Autodesk Fusion 360 part; units mm, degrees
(part 2 of 13)
  line L913 (104.217, -70.819) -> (104.221, -70.8155)
  line L914 (88.0199, -70.6373) -> (87.9134, -70.4952)
  line L915 (87.7957, -72.4288) -> (87.4385, -72.4288)
  line L916 (87.2885, -70.2788) -> (87.3086, -70.2038)
  line L917 (108.814, -71.9394) -> (108.833, -71.9473)
  line L918 (104.14, -72.3538) -> (104.085, -72.4087)
  line L919 (87.5885, -72.1288) -> (87.7639, -72.1288)
  line L920 (88.0792, -71.7621) -> (88.1457, -71.4077)
  line L921 (104.296, -70.7954) -> (104.439, -70.7954)
  line L922 (104.01, -70.7954) -> (104.085, -70.8155)
  line L923 (104.286, -70.7957) -> (104.291, -70.7967)
  line L924 (104.085, -72.4087) -> (104.01, -72.4288)
  line L925 (104.514, -71.0753) -> (104.439, -71.0954)
  line L926 (87.5885, -70.4288) -> (87.5885, -72.1288)
  line L927 (88.1457, -71.1498) -> (88.0792, -70.7954)
  line L928 (104.221, -70.8155) -> (104.254, -70.8067)
  line L929 (87.3086, -72.3538) -> (87.2885, -72.2788)
  line L930 (104.257, -71.1512) -> (104.214, -71.2087)
  line L931 (104.214, -71.2087) -> (104.16, -71.3536)
  line L932 (87.4385, -72.4288) -> (87.3635, -72.4087)
  line L933 (104.139, -70.8696) -> (104.212, -70.8206)
  line L934 (108.805, -71.9407) -> (108.814, -71.9394)
  line L935 (87.3086, -70.2038) -> (87.3635, -70.1489)
  line L936 (108.886, -71.9683) -> (108.899, -71.9851)
  line L937 (108.899, -71.9851) -> (108.916, -71.9983)
  line L938 (108.987, -72.0935) -> (108.994, -72.1103)
  line L939 (87.4385, -70.1288) -> (87.7957, -70.1288)
  line L940 (88.2808, -72.0632) -> (88.2728, -72.083)
  line L941 (88.1457, -71.4077) -> (88.1457, -71.1498)
  line L942 (104.439, -71.0954) -> (104.341, -71.0954)
  line L943 (88.0199, -71.9202) -> (88.0792, -71.7621)
  line L944 (87.8566, -72.4158) -> (87.8258, -72.4207)
  line L945 (87.7957, -70.1288) -> (87.8258, -70.1368)
  line L946 (103.371, -70.8155) -> (103.426, -70.8704)
  line L947 (102.792, -72.4087) -> (102.789, -72.4052)
  line L948 (103.371, -72.4087) -> (103.296, -72.4288)
  line L949 (108.814, -72.4277) -> (108.805, -72.4264)
  line L950 (108.73, -71.956) -> (108.737, -71.9503)
  line L951 (108.877, -71.9649) -> (108.886, -71.9683)
  line L952 (108.758, -71.9473) -> (108.778, -71.9394)
  line L953 (108.778, -71.9394) -> (108.787, -71.9407)
  line L954 (109.008, -72.2213) -> (109.005, -72.2424)
  line L955 (108.604, -72.2735) -> (108.598, -72.2567)
  line L956 (108.721, -71.9584) -> (108.73, -71.956)
  line L957 (108.598, -72.1103) -> (108.604, -72.0935)
  line L958 (102.611, -72.2737) -> (102.59, -72.25)
  line L959 (108.871, -71.9584) -> (108.877, -71.9649)
  line L960 (108.787, -72.4264) -> (108.778, -72.4277)
  line L961 (108.787, -71.9407) -> (108.796, -71.9383)
  line L962 (108.604, -72.0935) -> (108.676, -71.9983)
  line L963 (108.586, -72.1246) -> (108.598, -72.1103)
  line L964 (109.005, -72.2424) -> (108.994, -72.2567)
  line L965 (108.862, -72.411) -> (108.855, -72.4167)
  line L966 (109.016, -72.2015) -> (109.008, -72.2213)
  line L967 (103.426, -70.8704) -> (103.446, -70.9454)
  line L968 (108.692, -72.382) -> (108.676, -72.3688)
  line L969 (108.586, -72.2424) -> (108.583, -72.2213)
  line L970 (108.833, -72.4197) -> (108.814, -72.4277)
  line L971 (108.862, -71.956) -> (108.871, -71.9584)
  line L972 (108.583, -72.2213) -> (108.575, -72.2015)
  line L973 (108.758, -72.4197) -> (108.737, -72.4167)
  line L974 (108.598, -72.2567) -> (108.586, -72.2424)
  line L975 (108.737, -71.9503) -> (108.758, -71.9473)
  line L976 (109.005, -72.1246) -> (109.008, -72.1458)
  line L977 (108.916, -71.9983) -> (108.987, -72.0935)
  line L978 (108.855, -72.4167) -> (108.833, -72.4197)
  line L979 (108.796, -72.4288) -> (108.787, -72.4264)
  line L980 (108.778, -72.4277) -> (108.758, -72.4197)
  line L981 (109.013, -72.1835) -> (109.016, -72.2015)
  line L982 (108.994, -72.2567) -> (108.987, -72.2735)
  line L983 (108.871, -72.4087) -> (108.862, -72.411)
  line L984 (108.721, -72.4087) -> (108.714, -72.4022)
  line L985 (108.706, -72.3988) -> (108.692, -72.382)
  line L986 (108.676, -71.9983) -> (108.692, -71.9851)
  line L987 (108.575, -72.1656) -> (108.583, -72.1458)
  line L988 (108.796, -71.9383) -> (108.805, -71.9407)
  line L989 (108.994, -72.1103) -> (109.005, -72.1246)
  line L990 (108.877, -72.4022) -> (108.871, -72.4087)
  line L991 (108.676, -72.3688) -> (108.604, -72.2735)
  line L992 (108.583, -72.1458) -> (108.586, -72.1246)
  line L993 (108.805, -72.4264) -> (108.796, -72.4288)
  line L994 (109.016, -72.1656) -> (109.013, -72.1835)
  line L995 (108.916, -72.3688) -> (108.899, -72.382)
  line L996 (108.855, -71.9503) -> (108.862, -71.956)
  line L997 (108.692, -71.9851) -> (108.706, -71.9683)
  line L998 (109.008, -72.1458) -> (109.016, -72.1656)
  line L999 (108.833, -71.9473) -> (108.855, -71.9503)
  line L1000 (108.706, -71.9683) -> (108.714, -71.9649)
  line L1001 (108.886, -72.3988) -> (108.877, -72.4022)
  line L1002 (108.714, -71.9649) -> (108.721, -71.9584)
  line L1003 (108.899, -72.382) -> (108.886, -72.3988)
  line L1004 (108.987, -72.2735) -> (108.916, -72.3688)
  line L1005 (108.575, -72.2015) -> (108.578, -72.1835)
  line L1006 (108.578, -72.1835) -> (108.575, -72.1656)
  line L1007 (108.73, -72.411) -> (108.721, -72.4087)
  line L1008 (108.737, -72.4167) -> (108.73, -72.411)
  line L1009 (108.714, -72.4022) -> (108.706, -72.3988)
  line L1010 (133.278, -90.9545) -> (133.338, -90.8098)
  line L1011 (135.594, -81.6495) -> (135.593, -81.6559)
  line L1012 (134.438, -90.9545) -> (134.458, -91.1098)
  line L1013 (133.963, -83.4223) -> (133.964, -83.425)
  line L1014 (133.606, -83.3536) -> (133.61, -83.3452)
  line L1015 (133.631, -83.2877) -> (133.638, -83.2823)
  line L1016 (135.348, -72.6427) -> (135.292, -72.6351)
  line L1017 (135.596, -81.647) -> (135.594, -81.6495)
  line L1018 (135.562, -81.7087) -> (133.908, -83.3628)
  line L1019 (133.61, -83.3452) -> (133.609, -83.3362)
  line L1020 (133.946, -83.4014) -> (133.96, -83.4192)
  line L1021 (133.858, -91.7098) -> (133.703, -91.6894)
  line L1022 (134.158, -91.6294) -> (134.013, -91.6894)
  line L1023 (134.892, -71.4334) -> (135.012, -71.3164)
  line L1024 (133.558, -91.6294) -> (133.434, -91.5341)
  line L1025 (133.908, -83.3628) -> (133.946, -83.4014)
  line L1026 (106.922, -87.5998) -> (106.862, -87.4551)
  line L1027 (133.278, -91.2651) -> (133.258, -91.1098)
  line L1028 (133.338, -91.4098) -> (133.278, -91.2651)
  line L1029 (135.598, -72.6444) -> (135.598, -81.6204)
  line L1030 (133.619, -83.4136) -> (133.614, -83.4064)
  line L1031 (133.733, -83.5416) -> (133.643, -83.4512)
  line L1032 (133.643, -83.4512) -> (133.621, -83.4224)
  line L1033 (134.013, -91.6894) -> (133.858, -91.7098)
  line L1034 (108.022, -87.1445) -> (108.042, -87.2998)
  line L1035 (106.862, -87.4551) -> (106.842, -87.2998)
  line L1036 (135.577, -81.6817) -> (135.562, -81.7087)
  line L1037 (134.378, -91.4098) -> (134.282, -91.5341)
  line L1038 (133.434, -91.5341) -> (133.338, -91.4098)
  line L1039 (133.338, -90.8098) -> (133.434, -90.6855)
  line L1040 (107.142, -87.8194) -> (107.018, -87.7241)
  line L1041 (135.154, -71.2288) -> (135.312, -71.1749)
  line L1042 (133.643, -83.2744) -> (135.348, -81.5686)
  line L1043 (134.438, -91.2651) -> (134.378, -91.4098)
  line L1044 (133.258, -91.1098) -> (133.278, -90.9545)
  line L1045 (133.96, -83.4192) -> (133.963, -83.4223)
  line L1046 (135.624, -72.6421) -> (135.598, -72.6444)
  line L1047 (133.622, -83.3127) -> (133.631, -83.2877)
  line L1048 (133.983, -90.5263) -> (134.013, -90.5302)
  line L1049 (135.783, -72.5904) -> (135.624, -72.6421)
  line L1050 (133.612, -83.3797) -> (133.606, -83.3536)
  line L1051 (134.378, -90.8098) -> (134.438, -90.9545)
  line L1052 (133.434, -90.6855) -> (133.558, -90.5902)
  line L1053 (133.609, -83.3362) -> (133.622, -83.3127)
  line L1054 (133.638, -83.2823) -> (133.643, -83.2744)
  line L1055 (133.558, -90.5902) -> (133.703, -90.5302)
  line L1056 (134.282, -91.5341) -> (134.158, -91.6294)
  line L1057 (135.292, -72.6351) -> (135.135, -72.5768)
  line L1058 (108.022, -87.4551) -> (107.962, -87.5998)
  line L1059 (107.742, -87.8194) -> (107.597, -87.8794)
  line L1060 (133.703, -91.6894) -> (133.558, -91.6294)
  line L1061 (133.964, -83.425) -> (133.968, -83.4302)
  line L1062 (133.614, -83.4064) -> (133.612, -83.3797)
  line L1063 (135.348, -81.5686) -> (135.348, -72.6427)
  line L1064 (108.042, -87.2998) -> (108.022, -87.4551)
  line L1065 (107.442, -87.8998) -> (107.287, -87.8794)
  line L1066 (135.312, -71.1749) -> (135.479, -71.1574)
  line L1067 (133.733, -90.5263) -> (133.733, -83.5416)
  line L1068 (133.621, -83.4224) -> (133.619, -83.4136)
  line L1069 (135.012, -71.3164) -> (135.154, -71.2288)
  line L1070 (134.74, -72.0633) -> (134.724, -71.8969)
  line L1071 (136.048, -72.3895) -> (135.927, -72.5048)
  line L1072 (136.2, -72.0939) -> (136.141, -72.2502)
  line L1073 (133.703, -90.5302) -> (133.733, -90.5263)
  line L1074 (107.866, -87.7241) -> (107.742, -87.8194)
  line L1075 (134.995, -72.4853) -> (134.879, -72.365)
  line L1076 (106.842, -87.2998) -> (106.862, -87.1445)
  line L1077 (128.608, -80.6108) -> (128.615, -80.6409)
  line L1078 (120.961, -72.2502) -> (120.869, -72.3895)
  line L1079 (107.597, -86.7202) -> (107.742, -86.7802)
  line L1080 (111.956, -87.6733) -> (111.831, -87.7686)
  line L1081 (120.764, -71.3229) -> (120.882, -71.4415)
  line L1082 (112.131, -87.249) -> (112.111, -87.4043)
  line L1083 (111.231, -86.7294) -> (111.376, -86.6694)
  line L1084 (107.018, -86.8755) -> (107.142, -86.7802)
  line L1085 (111.956, -86.8247) -> (112.051, -86.949)
  line L1086 (112.051, -87.549) -> (111.956, -87.6733)
  line L1087 (107.597, -87.8794) -> (107.442, -87.8998)
  line L1088 (106.862, -87.1445) -> (106.922, -86.9998)
  line L1089 (110.931, -87.249) -> (110.952, -87.0937)
  line L1090 (107.287, -87.8794) -> (107.142, -87.8194)
  line L1091 (106.922, -86.9998) -> (107.018, -86.8755)
  line L1092 (111.531, -87.849) -> (111.376, -87.8286)
  line L1093 (120.623, -71.2333) -> (120.764, -71.3229)
  line L1094 (111.107, -87.6733) -> (111.012, -87.549)
  line L1095 (112.111, -87.4043) -> (112.051, -87.549)
  line L1096 (107.962, -86.9998) -> (108.022, -87.1445)
  line L1097 (107.287, -86.7202) -> (107.442, -86.6998)
  line L1098 (112.111, -87.0937) -> (112.131, -87.249)
  line L1099 (107.742, -86.7802) -> (107.866, -86.8755)
  line L1100 (107.018, -87.7241) -> (106.922, -87.5998)
  line L1101 (135.135, -72.5768) -> (134.995, -72.4853)
  line L1102 (111.831, -87.7686) -> (111.687, -87.8286)
  line L1103 (120.466, -71.1772) -> (120.623, -71.2333)
  line L1104 (111.687, -87.8286) -> (111.531, -87.849)
  line L1105 (135.479, -71.1574) -> (135.645, -71.1772)
  line L1106 (107.866, -86.8755) -> (107.962, -86.9998)
  line L1107 (128.605, -80.6056) -> (128.608, -80.6108)
  line L1108 (128.615, -80.6409) -> (128.624, -80.6704)
  line L1109 (111.012, -86.949) -> (111.107, -86.8247)
  line L1110 (128.624, -86.7664) -> (128.621, -86.7846)
  line L1111 (128.621, -86.7846) -> (128.621, -86.7895)
  line L1112 (134.724, -71.8969) -> (134.744, -71.731)
  line L1113 (107.962, -87.5998) -> (107.866, -87.7241)
  line L1114 (111.376, -87.8286) -> (111.231, -87.7686)
  line L1115 (110.952, -87.0937) -> (111.012, -86.949)
  line L1116 (128.415, -87.0369) -> (128.447, -87.1)
  line L1117 (134.744, -71.731) -> (134.802, -71.5739)
  line L1118 (111.107, -86.8247) -> (111.231, -86.7294)
  line L1119 (111.831, -86.7294) -> (111.956, -86.8247)
  line L1120 (134.879, -72.365) -> (134.793, -72.222)
  line L1121 (112.051, -86.949) -> (112.111, -87.0937)
  line L1122 (107.142, -86.7802) -> (107.287, -86.7202)
  line L1123 (111.376, -86.6694) -> (111.531, -86.649)
  line L1124 (107.442, -86.6998) -> (107.597, -86.7202)
  line L1125 (128.447, -87.1) -> (128.467, -87.2236)
  line L1126 (128.621, -86.7895) -> (128.62, -86.7928)
  line L1127 (110.952, -87.4043) -> (110.931, -87.249)
  line L1128 (111.531, -86.649) -> (111.687, -86.6694)
  line L1129 (111.687, -86.6694) -> (111.831, -86.7294)
  line L1130 (128.467, -87.2236) -> (128.447, -87.3472)
  line L1131 (134.793, -72.222) -> (134.74, -72.0633)
  line L1132 (134.802, -71.5739) -> (134.892, -71.4334)
  line L1133 (111.012, -87.549) -> (110.952, -87.4043)
  line L1134 (128.603, -86.8263) -> (128.589, -86.8522)
  line L1135 (128.39, -87.4587) -> (128.302, -87.5472)
  line L1136 (111.231, -87.7686) -> (111.107, -87.6733)
  line L1137 (121.044, -71.9074) -> (121.044, -71.9283)
  line L1138 (120.604, -72.5904) -> (120.598, -72.5926)
  line L1139 (128.233, -86.8651) -> (128.374, -86.7167)
  line L1140 (95.5416, -85.8896) -> (95.5238, -85.9029)
  line L1141 (95.4532, -85.9262) -> (88.3145, -85.9262)
  line L1142 (127.139, -82.6056) -> (127.199, -82.7503)
  line L1143 (128.587, -80.582) -> (128.6, -80.5998)
  line L1144 (128.374, -86.7167) -> (128.374, -80.7222)
  line L1145 (88.309, -85.9779) -> (88.2541, -86.1469)
  line L1146 (119.975, -71.2288) -> (120.133, -71.1749)
  line L1147 (121.026, -71.7412) -> (121.044, -71.9074)
  line L1148 (128.62, -86.7928) -> (128.618, -86.8019)
  line L1149 (119.614, -72.222) -> (119.561, -72.0633)
  line L1150 (119.561, -72.0633) -> (119.544, -71.8969)
  line L1151 (128.19, -86.8432) -> (128.233, -86.8651)
  line L1152 (120.113, -72.6351) -> (119.956, -72.5768)
  line L1153 (128.6, -80.5998) -> (128.604, -80.6029)
  line L1154 (128.19, -87.604) -> (128.067, -87.6236)
  line L1155 (120.748, -72.5048) -> (120.604, -72.5904)
  line L1156 (127.686, -87.3472) -> (127.667, -87.2236)
  line L1157 (119.713, -71.4334) -> (119.833, -71.3164)
  line L1158 (128.374, -80.7222) -> (120.306, -72.6547)
  line L1159 (119.816, -72.4853) -> (119.7, -72.365)
  line L1160 (95.5207, -85.9064) -> (95.518, -85.9072)
  line L1161 (120.598, -72.5926) -> (128.587, -80.582)
  line L1162 (120.306, -72.6547) -> (120.279, -72.6572)
  line L1163 (127.943, -86.8432) -> (128.067, -86.8236)
  line L1164 (120.133, -71.1749) -> (120.3, -71.1574)
  line L1165 (119.7, -72.365) -> (119.614, -72.222)
  line L1166 (99.2673, -85.1301) -> (99.2378, -85.1388)
  line L1167 (128.067, -86.8236) -> (128.19, -86.8432)
  line L1168 (120.971, -71.5833) -> (121.026, -71.7412)
  line L1169 (88.3145, -85.9262) -> (88.309, -85.9779)
  line L1170 (121.021, -72.0939) -> (120.961, -72.2502)
  line L1171 (95.4827, -85.9175) -> (95.4532, -85.9262)
  line L1172 (128.302, -87.5472) -> (128.19, -87.604)
  line L1173 (127.943, -87.604) -> (127.832, -87.5472)
  line L1174 (127.043, -83.3299) -> (126.919, -83.4252)
  line L1175 (95.5128, -85.9111) -> (95.4827, -85.9175)
  line L1176 (99.3026, -85.1198) -> (99.2974, -85.1237)
  line L1177 (120.882, -71.4415) -> (120.971, -71.5833)
  line L1178 (127.832, -87.5472) -> (127.743, -87.4587)
  line L1179 (127.743, -86.9885) -> (127.832, -86.9)
  line L1180 (126.774, -82.326) -> (126.919, -82.386)
  line L1181 (120.3, -71.1574) -> (120.466, -71.1772)
  line L1182 (120.869, -72.3895) -> (120.748, -72.5048)
  line L1183 (99.2378, -85.1388) -> (96.2924, -85.1388)
  line L1184 (127.199, -82.7503) -> (127.219, -82.9056)
  line L1185 (121.044, -71.9283) -> (121.021, -72.0939)
  line L1186 (120.279, -72.6572) -> (120.113, -72.6351)
  line L1187 (128.604, -80.6029) -> (128.605, -80.6056)
  line L1188 (128.067, -87.6236) -> (127.943, -87.604)
  line L1189 (127.686, -87.1) -> (127.743, -86.9885)
  line L1190 (128.589, -86.8522) -> (128.415, -87.0369)
  line L1191 (127.743, -87.4587) -> (127.686, -87.3472)
  line L1192 (119.565, -71.731) -> (119.623, -71.5739)
  line L1193 (128.618, -86.8019) -> (128.603, -86.8263)
  line L1194 (119.956, -72.5768) -> (119.816, -72.4853)
  line L1195 (128.447, -87.3472) -> (128.39, -87.4587)
  line L1196 (119.833, -71.3164) -> (119.975, -71.2288)
  line L1197 (127.832, -86.9) -> (127.943, -86.8432)
  line L1198 (128.624, -80.6704) -> (128.624, -86.7664)
  line L1199 (127.667, -87.2236) -> (127.686, -87.1)
  line L1200 (119.544, -71.8969) -> (119.565, -71.731)
  line L1201 (119.623, -71.5739) -> (119.713, -71.4334)
  line L1202 (109.464, -86.0298) -> (109.444, -86.1851)
  line L1203 (87.2149, -84.9928) -> (87.3888, -84.9559)
  line L1204 (88.2541, -86.1469) -> (88.1653, -86.3008)
  line L1205 (126.774, -83.4852) -> (126.619, -83.5056)
  line L1206 (86.7899, -86.3008) -> (86.7011, -86.1469)
  line L1207 (87.7403, -86.6096) -> (87.5664, -86.6465)
  line L1208 (88.0464, -85.1695) -> (88.1653, -85.3016)
  line L1209 (87.5664, -86.6465) -> (87.3888, -86.6465)
  line L1210 (87.5664, -84.9559) -> (87.7403, -84.9928)
  line L1211 (100.938, -83.1413) -> (100.941, -83.1378)
  line L1212 (95.518, -85.9072) -> (95.5128, -85.9111)
  line L1213 (87.0526, -86.5373) -> (86.9088, -86.4329)
  line L1214 (99.2974, -85.1237) -> (99.2673, -85.1301)
  line L1215 (109.289, -86.4541) -> (109.164, -86.5494)
  line L1216 (96.1522, -84.9254) -> (96.17, -84.9121)
  line L1217 (86.7011, -85.4555) -> (86.7899, -85.3016)
  line L1218 (127.043, -82.4813) -> (127.139, -82.6056)
  line L1219 (96.2924, -85.1388) -> (95.5416, -85.8896)
  line L1220 (99.3262, -85.1022) -> (99.3084, -85.1155)
  line L1221 (86.6462, -85.9779) -> (86.6276, -85.8012)
  line L1222 (88.1653, -85.3016) -> (88.2541, -85.4555)
  line L1223 (95.4014, -85.6762) -> (96.1522, -84.9254)
  line L1224 (101.06, -83.368) -> (99.3262, -85.1022)
  line L1225 (109.444, -86.1851) -> (109.384, -86.3298)
  line L1226 (99.186, -84.8888) -> (100.92, -83.1546)
  line L1227 (109.164, -86.5494) -> (109.02, -86.6094)
  line L1228 (86.9088, -86.4329) -> (86.7899, -86.3008)
  line L1229 (126.919, -83.4252) -> (126.774, -83.4852)
  line L1230 (127.199, -83.0609) -> (127.139, -83.2056)
  line L1231 (126.244, -83.368) -> (101.06, -83.368)
  line L1232 (87.3888, -86.6465) -> (87.2149, -86.6096)
  line L1233 (88.2541, -85.4555) -> (88.309, -85.6245)
  line L1234 (86.6462, -85.6245) -> (86.7011, -85.4555)
  line L1235 (86.7011, -86.1469) -> (86.6462, -85.9779)
  line L1236 (87.3888, -84.9559) -> (87.5664, -84.9559)
  line L1237 (86.6276, -85.8012) -> (86.6462, -85.6245)
  line L1238 (86.9088, -85.1695) -> (87.0526, -85.0651)
  line L1239 (126.919, -82.386) -> (127.043, -82.4813)
  line L1240 (86.7899, -85.3016) -> (86.9088, -85.1695)
  line L1241 (87.7403, -84.9928) -> (87.9026, -85.0651)
  line L1242 (126.619, -83.5056) -> (126.464, -83.4852)
  line L1243 (87.2149, -86.6096) -> (87.0526, -86.5373)
  line L1244 (87.9026, -85.0651) -> (88.0464, -85.1695)
  line L1245 (88.3145, -85.6762) -> (95.4014, -85.6762)
  line L1246 (95.5238, -85.9029) -> (95.5207, -85.9064)
  line L1247 (96.17, -84.9121) -> (96.1731, -84.9086)
  line L1248 (127.219, -82.9056) -> (127.199, -83.0609)
  line L1249 (127.139, -83.2056) -> (127.043, -83.3299)
  line L1250 (126.464, -83.4852) -> (126.319, -83.4252)
  line L1251 (99.3053, -85.119) -> (99.3026, -85.1198)
  line L1252 (126.319, -83.4252) -> (126.244, -83.368)
  line L1253 (87.9026, -86.5373) -> (87.7403, -86.6096)
  line L1254 (88.0464, -86.4329) -> (87.9026, -86.5373)
  line L1255 (88.309, -85.6245) -> (88.3145, -85.6762)
  line L1256 (100.92, -83.1546) -> (100.938, -83.1413)
  line L1257 (126.464, -82.326) -> (126.619, -82.3056)
  line L1258 (101.009, -83.118) -> (126.063, -83.118)
  line L1259 (99.3084, -85.1155) -> (99.3053, -85.119)
  line L1260 (126.619, -82.3056) -> (126.774, -82.326)
  line L1261 (96.181, -84.9039) -> (96.2111, -84.8975)
  line L1262 (109.384, -86.3298) -> (109.289, -86.4541)
  line L1263 (88.1653, -86.3008) -> (88.0464, -86.4329)
  line L1264 (87.0526, -85.0651) -> (87.2149, -84.9928)
  line L1265 (100.949, -83.1331) -> (100.979, -83.1267)
  line L1266 (108.042, -84.6836) -> (108.022, -84.8389)
  line L1267 (107.597, -85.2632) -> (107.442, -85.2836)
  line L1268 (126.019, -82.9056) -> (126.039, -82.7503)
  line L1269 (96.2406, -84.8888) -> (99.186, -84.8888)
  line L1270 (126.039, -83.0609) -> (126.019, -82.9056)
  line L1271 (96.1758, -84.9078) -> (96.181, -84.9039)
  line L1272 (96.1731, -84.9086) -> (96.1758, -84.9078)
  line L1273 (96.2111, -84.8975) -> (96.2406, -84.8888)
  line L1274 (109.02, -85.4502) -> (109.164, -85.5102)
  line L1275 (100.941, -83.1378) -> (100.944, -83.137)
  line L1276 (109.164, -85.5102) -> (109.289, -85.6055)
  line L1277 (126.319, -82.386) -> (126.464, -82.326)
  line L1278 (107.287, -85.2632) -> (107.142, -85.2032)
  line L1279 (108.022, -84.5283) -> (108.042, -84.6836)
  line L1280 (109.289, -85.6055) -> (109.384, -85.7298)
  line L1281 (108.44, -86.4541) -> (108.345, -86.3298)
  line L1282 (108.709, -85.4502) -> (108.864, -85.4298)
  line L1283 (107.442, -85.2836) -> (107.287, -85.2632)
  line L1284 (109.444, -85.8745) -> (109.464, -86.0298)
  line L1285 (100.979, -83.1267) -> (101.009, -83.118)
  line L1286 (107.962, -84.3836) -> (108.022, -84.5283)
  line L1287 (108.345, -85.7298) -> (108.44, -85.6055)
  line L1288 (126.039, -82.7503) -> (126.099, -82.6056)
  line L1289 (126.195, -82.4813) -> (126.319, -82.386)
  line L1290 (106.922, -84.9836) -> (106.862, -84.8389)
  line L1291 (107.018, -85.1079) -> (106.922, -84.9836)
  line L1292 (108.864, -86.6298) -> (108.709, -86.6094)
  line L1293 (108.345, -86.3298) -> (108.285, -86.1851)
  line L1294 (109.384, -85.7298) -> (109.444, -85.8745)
  line L1295 (126.099, -82.6056) -> (126.195, -82.4813)
  line L1296 (107.597, -84.104) -> (107.742, -84.164)
  line L1297 (108.709, -86.6094) -> (108.564, -86.5494)
  line L1298 (107.866, -85.1079) -> (107.742, -85.2032)
  line L1299 (100.944, -83.137) -> (100.949, -83.1331)
  line L1300 (126.063, -83.118) -> (126.039, -83.0609)
  line L1301 (106.842, -84.6836) -> (106.862, -84.5283)
  line L1302 (108.44, -85.6055) -> (108.564, -85.5102)
  line L1303 (108.564, -86.5494) -> (108.44, -86.4541)
  line L1304 (108.285, -86.1851) -> (108.264, -86.0298)
  line L1305 (106.862, -84.8389) -> (106.842, -84.6836)
  line L1306 (107.866, -84.2593) -> (107.962, -84.3836)
  line L1307 (107.142, -85.2032) -> (107.018, -85.1079)
  line L1308 (108.564, -85.5102) -> (108.709, -85.4502)
  line L1309 (107.742, -84.164) -> (107.866, -84.2593)
  line L1310 (87.7403, -84.0696) -> (87.5664, -84.1065)
  line L1311 (107.018, -84.2593) -> (107.142, -84.164)
  line L1312 (109.388, -82.0928) -> (109.368, -82.2481)
  line L1313 (108.364, -81.6685) -> (108.488, -81.5732)
  line L1314 (108.285, -85.8745) -> (108.345, -85.7298)
  line L1315 (86.7011, -82.9155) -> (86.7899, -82.7616)
  line L1316 (87.9026, -83.9973) -> (87.7403, -84.0696)
  line L1317 (108.022, -84.8389) -> (107.962, -84.9836)
  line L1318 (86.7011, -83.6069) -> (86.6462, -83.4379)
  line L1319 (87.2149, -84.0696) -> (87.0526, -83.9973)
  line L1320 (109.02, -86.6094) -> (108.864, -86.6298)
  line L1321 (86.7899, -83.7608) -> (86.7011, -83.6069)
  line L1322 (107.287, -84.104) -> (107.442, -84.0836)
  line L1323 (107.142, -84.164) -> (107.287, -84.104)
  line L1324 (107.442, -84.0836) -> (107.597, -84.104)
  line L1325 (88.2541, -82.9155) -> (88.309, -83.0845)
  line L1326 (109.212, -81.6685) -> (109.308, -81.7928)
  line L1327 (86.9088, -82.6295) -> (87.0526, -82.5251)
  line L1328 (88.2541, -83.6069) -> (88.1653, -83.7608)
  line L1329 (109.308, -81.7928) -> (109.368, -81.9375)
  line L1330 (88.1653, -82.7616) -> (88.2541, -82.9155)
  line L1331 (86.6276, -83.2612) -> (86.6462, -83.0845)
  line L1332 (88.3276, -83.2612) -> (88.309, -83.4379)
  line L1333 (108.864, -85.4298) -> (109.02, -85.4502)
  line L1334 (88.309, -83.0845) -> (88.3276, -83.2612)
  line L1335 (109.088, -81.5732) -> (109.212, -81.6685)
  line L1336 (88.1653, -83.7608) -> (88.0464, -83.8929)
  line L1337 (88.0464, -82.6295) -> (88.1653, -82.7616)
  line L1338 (106.862, -84.5283) -> (106.922, -84.3836)
  line L1339 (86.7899, -82.7616) -> (86.9088, -82.6295)
  line L1340 (87.0526, -83.9973) -> (86.9088, -83.8929)
  line L1341 (109.368, -82.2481) -> (109.308, -82.3928)
  line L1342 (107.742, -85.2032) -> (107.597, -85.2632)
  line L1343 (88.309, -83.4379) -> (88.2541, -83.6069)
  line L1344 (86.6462, -83.4379) -> (86.6276, -83.2612)
  line L1345 (87.9026, -82.5251) -> (88.0464, -82.6295)
  line L1346 (87.5664, -84.1065) -> (87.3888, -84.1065)
  line L1347 (86.6462, -83.0845) -> (86.7011, -82.9155)
  line L1348 (86.9088, -83.8929) -> (86.7899, -83.7608)
  line L1349 (88.0464, -83.8929) -> (87.9026, -83.9973)
  line L1350 (107.962, -84.9836) -> (107.866, -85.1079)
  line L1351 (87.7403, -82.4528) -> (87.9026, -82.5251)
  line L1352 (106.922, -84.3836) -> (107.018, -84.2593)
  line L1353 (108.264, -86.0298) -> (108.285, -85.8745)
  line L1354 (87.3888, -84.1065) -> (87.2149, -84.0696)
  line L1355 (108.943, -82.6724) -> (108.788, -82.6928)
  line L1356 (124.214, -82.0853) -> (124.118, -81.961)
  line L1357 (124.938, -81.1414) -> (125.062, -81.2367)
  line L1358 (124.038, -81.661) -> (124.058, -81.5057)
  line L1359 (124.214, -81.2367) -> (124.338, -81.1414)
  line L1360 (122.624, -82.0091) -> (122.499, -82.1044)
  line L1361 (124.938, -82.1806) -> (124.793, -82.2406)
  line L1362 (108.188, -82.0928) -> (108.209, -81.9375)
  line L1363 (87.0526, -82.5251) -> (87.2149, -82.4528)
  line L1364 (122.719, -81.2848) -> (122.779, -81.4295)
  line L1365 (125.238, -81.661) -> (125.217, -81.8163)
  line L1366 (124.338, -82.1806) -> (124.214, -82.0853)
  line L1367 (124.793, -82.2406) -> (124.638, -82.261)
  line L1368 (124.793, -81.0814) -> (124.938, -81.1414)
  line L1369 (125.157, -81.361) -> (125.217, -81.5057)
  line L1370 (108.488, -82.6124) -> (108.364, -82.5171)
  line L1371 (109.308, -82.3928) -> (109.212, -82.5171)
  line L1372 (122.499, -82.1044) -> (122.355, -82.1644)
  line L1373 (125.157, -81.961) -> (125.062, -82.0853)
  line L1374 (124.338, -81.1414) -> (124.483, -81.0814)
  line L1375 (122.044, -82.1644) -> (121.899, -82.1044)
  line L1376 (108.269, -82.3928) -> (108.209, -82.2481)
  line L1377 (122.624, -81.1605) -> (122.719, -81.2848)
  line L1378 (108.788, -81.4928) -> (108.943, -81.5132)
  line L1379 (125.217, -81.8163) -> (125.157, -81.961)
  line L1380 (109.088, -82.6124) -> (108.943, -82.6724)
  line L1381 (125.217, -81.5057) -> (125.238, -81.661)
  line L1382 (124.483, -81.0814) -> (124.638, -81.061)
  line L1383 (124.638, -81.061) -> (124.793, -81.0814)
  line L1384 (122.779, -81.7401) -> (122.719, -81.8848)
  line L1385 (108.943, -81.5132) -> (109.088, -81.5732)
  line L1386 (108.364, -82.5171) -> (108.269, -82.3928)
  line L1387 (125.062, -81.2367) -> (125.157, -81.361)
  line L1388 (108.209, -82.2481) -> (108.188, -82.0928)
  line L1389 (87.5664, -82.4159) -> (87.7403, -82.4528)
  line L1390 (121.68, -81.2848) -> (121.775, -81.1605)
  line L1391 (92.9829, -80.5244) -> (93.1404, -80.5805)
  line L1392 (124.483, -82.2406) -> (124.338, -82.1806)
  line L1393 (108.269, -81.7928) -> (108.364, -81.6685)
  line L1394 (108.488, -81.5732) -> (108.633, -81.5132)
  line L1395 (122.355, -81.0052) -> (122.499, -81.0652)
  line L1396 (108.209, -81.9375) -> (108.269, -81.7928)
  line L1397 (87.3888, -82.4159) -> (87.5664, -82.4159)
  line L1398 (109.212, -82.5171) -> (109.088, -82.6124)
  line L1399 (87.2149, -82.4528) -> (87.3888, -82.4159)
  line L1400 (122.799, -81.5848) -> (122.779, -81.7401)
  line L1401 (122.355, -82.1644) -> (122.199, -82.1848)
  line L1402 (108.633, -81.5132) -> (108.788, -81.4928)
  line L1403 (124.058, -81.8163) -> (124.038, -81.661)
  line L1404 (122.199, -82.1848) -> (122.044, -82.1644)
  line L1405 (124.118, -81.361) -> (124.214, -81.2367)
  line L1406 (124.058, -81.5057) -> (124.118, -81.361)
  line L1407 (122.779, -81.4295) -> (122.799, -81.5848)
  line L1408 (124.118, -81.961) -> (124.058, -81.8163)
  line L1409 (122.499, -81.0652) -> (122.624, -81.1605)
  line L1410 (125.062, -82.0853) -> (124.938, -82.1806)
  line L1411 (108.788, -82.6928) -> (108.633, -82.6724)
  line L1412 (109.368, -81.9375) -> (109.388, -82.0928)
  line L1413 (122.719, -81.8848) -> (122.624, -82.0091)
  line L1414 (108.633, -82.6724) -> (108.488, -82.6124)
  line L1415 (124.638, -82.261) -> (124.483, -82.2406)
  line L1416 (92.0826, -81.0782) -> (92.1398, -80.9211)
  line L1417 (121.899, -82.1044) -> (121.775, -82.0091)
  line L1418 (121.775, -81.1605) -> (121.899, -81.0652)
  line L1419 (92.6302, -81.9823) -> (92.4734, -81.924)
  line L1420 (92.2174, -81.7122) -> (92.1308, -81.5692)
  line L1421 (122.199, -80.9848) -> (122.355, -81.0052)
  line L1422 (121.68, -81.8848) -> (121.62, -81.7401)
  line L1423 (115.984, -71.9283) -> (115.961, -72.0939)
  line L1424 (93.5613, -81.2755) -> (93.538, -81.4411)
  line L1425 (92.1398, -80.9211) -> (92.2304, -80.7806)
  line L1426 (121.62, -81.4295) -> (121.68, -81.2848)
  line L1427 (121.899, -81.0652) -> (122.044, -81.0052)
  line L1428 (115.985, -71.9074) -> (115.984, -71.9283)
  line L1429 (86.6276, -81.5712) -> (86.6276, -79.8712)
  line L1430 (115.966, -71.7412) -> (115.985, -71.9074)
  line L1431 (92.3499, -80.6636) -> (92.4923, -80.576)
  line L1432 (92.0617, -81.2441) -> (92.0826, -81.0782)
  line L1433 (88.3276, -81.5712) -> (86.6276, -81.5712)
  line L1434 (115.705, -71.3229) -> (115.822, -71.4415)
  line L1435 (115.902, -72.2502) -> (115.809, -72.3895)
  line L1436 (92.6505, -80.5221) -> (92.8168, -80.5046)
  line L1437 (115.809, -72.3895) -> (115.688, -72.5048)
  line L1438 (121.62, -81.7401) -> (121.599, -81.5848)
  line L1439 (92.7959, -82.0044) -> (92.6302, -81.9823)
  line L1440 (88.3276, -79.8712) -> (88.3276, -81.5712)
  line L1441 (115.961, -72.0939) -> (115.902, -72.2502)
  line L1442 (122.044, -81.0052) -> (122.199, -80.9848)
  line L1443 (93.538, -81.4411) -> (93.4787, -81.5974)
  line L1444 (93.488, -80.9305) -> (93.543, -81.0884)
  line L1445 (93.3861, -81.7367) -> (93.265, -81.852)
  line L1446 (93.265, -81.852) -> (93.1214, -81.9376)
  line L1447 (93.4787, -81.5974) -> (93.3861, -81.7367)
  line L1448 (121.775, -82.0091) -> (121.68, -81.8848)
  line L1449 (93.1404, -80.5805) -> (93.2816, -80.6701)
  line L1450 (93.5616, -81.2546) -> (93.5613, -81.2755)
  line L1451 (93.1214, -81.9376) -> (92.9624, -81.9893)
  line L1452 (93.3994, -80.7887) -> (93.488, -80.9305)
  line L1453 (92.4734, -81.924) -> (92.3335, -81.8325)
  line L1454 (92.3335, -81.8325) -> (92.2174, -81.7122)
  line L1455 (92.1308, -81.5692) -> (92.078, -81.4105)
  line L1456 (86.6276, -79.8712) -> (88.3276, -79.8712)
  line L1457 (115.386, -72.6421) -> (115.219, -72.6572)
  line L1458 (115.053, -72.6351) -> (114.897, -72.5768)
  line L1459 (92.2304, -80.7806) -> (92.3499, -80.6636)
  line L1460 (114.757, -72.4853) -> (114.641, -72.365)
  line L1461 (93.543, -81.0884) -> (93.5616, -81.2546)
  line L1462 (92.9624, -81.9893) -> (92.7959, -82.0044)
  line L1463 (115.822, -71.4415) -> (115.911, -71.5833)
  line L1464 (115.911, -71.5833) -> (115.966, -71.7412)
  line L1465 (115.219, -72.6572) -> (115.053, -72.6351)
  line L1466 (115.688, -72.5048) -> (115.545, -72.5904)
  line L1467 (114.641, -72.365) -> (114.554, -72.222)
  line L1468 (92.078, -81.4105) -> (92.0617, -81.2441)
  line L1469 (93.2816, -80.6701) -> (93.3994, -80.7887)
  line L1470 (121.599, -81.5848) -> (121.62, -81.4295)
  line L1471 (115.406, -71.1772) -> (115.563, -71.2333)
  line L1472 (114.897, -72.5768) -> (114.757, -72.4853)
  line L1473 (115.545, -72.5904) -> (115.386, -72.6421)
  line L1474 (92.4923, -80.576) -> (92.6505, -80.5221)
  line L1475 (92.8168, -80.5046) -> (92.9829, -80.5244)
  line L1476 (115.563, -71.2333) -> (115.705, -71.3229)
  line L1477 (92.6504, -71.2737) -> (92.653, -71.3004)
  line L1478 (114.554, -72.222) -> (114.501, -72.0633)
  line L1479 (92.579, -71.0832) -> (92.6504, -71.2737)
  line L1480 (92.2663, -70.8067) -> (92.2993, -70.8155)
  line L1481 (92.6504, -71.9505) -> (92.579, -72.141)
  line L1482 (92.2993, -70.8155) -> (92.3028, -70.819)
  line L1483 (114.915, -71.2288) -> (115.074, -71.1749)
  line L1484 (92.3028, -70.819) -> (92.3075, -70.8206)
  line L1485 (92.5665, -71.0658) -> (92.579, -71.0832)
  line L1486 (92.579, -72.141) -> (92.5665, -72.1584)
  line L1487 (92.2339, -70.7957) -> (92.2663, -70.8067)
  line L1488 (114.501, -72.0633) -> (114.485, -71.8969)
  line L1489 (92.66, -71.8978) -> (92.653, -71.9238)
  line L1490 (92.5665, -72.1584) -> (92.5585, -72.1783)
  line L1491 (115.074, -71.1749) -> (115.24, -71.1574)
  line L1492 (92.4871, -72.2735) -> (92.4671, -72.2892)
  line L1493 (92.3075, -70.8206) -> (92.4503, -70.9159)
  line L1494 (114.654, -71.4334) -> (114.773, -71.3164)
  line L1495 (92.653, -71.3004) -> (92.66, -71.3264)
  line L1496 (92.653, -71.9238) -> (92.6504, -71.9505)
  line L1497 (92.66, -71.3264) -> (92.66, -71.8978)
  line L1498 (92.5585, -72.1783) -> (92.4871, -72.2735)
  line L1499 (114.773, -71.3164) -> (114.915, -71.2288)
  line L1500 (91.5812, -71.3004) -> (91.5838, -71.2737)
  line L1501 (91.5838, -71.2737) -> (91.6552, -71.0832)
  line L1502 (92.01, -72.4288) -> (92.0052, -72.4275)
  line L1503 (91.5743, -71.8978) -> (91.5743, -71.3264)
  line L1504 (91.6757, -72.1783) -> (91.6677, -72.1584)
  line L1505 (91.7471, -70.9507) -> (91.7671, -70.935)
  line L1506 (91.6757, -71.0459) -> (91.7471, -70.9507)
  line L1507 (114.485, -71.8969) -> (114.506, -71.731)
  line L1508 (91.6677, -71.0658) -> (91.6757, -71.0459)
  line L1509 (91.9315, -72.4052) -> (91.9268, -72.4036)
  line L1510 (92.4671, -70.935) -> (92.4871, -70.9507)
  line L1511 (91.935, -72.4087) -> (91.9315, -72.4052)
  line L1512 (91.6552, -71.0832) -> (91.6677, -71.0658)
  line L1513 (92.4503, -72.3083) -> (92.3075, -72.4036)
  line L1514 (92.229, -72.4275) -> (92.2243, -72.4288)
  line L1515 (91.968, -72.4175) -> (91.935, -72.4087)
  line L1516 (91.6552, -72.141) -> (91.5838, -71.9505)
  line L1517 (114.506, -71.731) -> (114.563, -71.5739)
  line L1518 (92.4871, -70.9507) -> (92.5585, -71.0459)
  line L1519 (115.24, -71.1574) -> (115.406, -71.1772)
  line L1520 (92.5585, -71.0459) -> (92.5665, -71.0658)
  line L1521 (91.7839, -72.3083) -> (91.7671, -72.2892)
  line L1522 (91.5838, -71.9505) -> (91.5812, -71.9238)
  line L1523 (91.5812, -71.9238) -> (91.5743, -71.8978)
  line L1524 (92.4671, -72.2892) -> (92.4503, -72.3083)
  line L1525 (92.2993, -72.4087) -> (92.2663, -72.4175)
  line L1526 (91.9268, -72.4036) -> (91.7839, -72.3083)
  line L1527 (91.5743, -71.3264) -> (91.5812, -71.3004)
  line L1528 (92.3028, -72.4052) -> (92.2993, -72.4087)
  line L1529 (91.7671, -72.2892) -> (91.7471, -72.2735)
  line L1530 (91.7471, -72.2735) -> (91.6757, -72.1783)
  line L1531 (114.563, -71.5739) -> (114.654, -71.4334)
  line L1532 (92.2339, -72.4284) -> (92.229, -72.4275)
  line L1533 (91.6677, -72.1584) -> (91.6552, -72.141)
  line L1534 (92.4503, -70.9159) -> (92.4671, -70.935)
  line L1535 (92.229, -70.7967) -> (92.2339, -70.7957)
  line L1536 (92.0052, -72.4275) -> (92.0003, -72.4284)
  line L1537 (92.2243, -72.4288) -> (92.01, -72.4288)
  line L1538 (105.724, -71.2052) -> (105.731, -71.2311)
  line L1539 (92.0554, -71.0954) -> (91.9717, -71.1512)
  line L1540 (91.968, -70.8067) -> (92.0003, -70.7957)
  line L1541 (91.935, -70.8155) -> (91.968, -70.8067)
  line L1542 (105.67, -71.5376) -> (105.656, -71.5515)
  line L1543 (105.017, -71.7273) -> (105.017, -71.9658)
  line L1544 (92.2625, -71.1512) -> (92.1788, -71.0954)
  line L1545 (92.01, -70.7954) -> (92.2243, -70.7954)
  line L1546 (92.0003, -70.7957) -> (92.0052, -70.7967)
  line L1547 (91.8743, -71.3536) -> (91.8743, -71.8706)
  line L1548 (105.409, -70.8067) -> (105.442, -70.8155)
  line L1549 (105.446, -70.819) -> (105.45, -70.8206)
  line L1550 (92.3056, -72.0155) -> (92.36, -71.8706)
  line L1551 (105.731, -71.4216) -> (105.726, -71.4408)
  line L1552 (105.716, -71.4776) -> (105.711, -71.4966)
  line L1553 (92.3056, -71.2087) -> (92.2625, -71.1512)
  line L1554 (92.2625, -72.073) -> (92.3056, -72.0155)
  line L1555 (92.1788, -71.0954) -> (92.0554, -71.0954)
  line L1556 (92.2663, -72.4175) -> (92.2339, -72.4284)
  line L1557 (92.3075, -72.4036) -> (92.3028, -72.4052)
  line L1558 (92.0554, -72.1288) -> (92.1788, -72.1288)
  line L1559 (91.9717, -72.073) -> (92.0554, -72.1288)
  line L1560 (105.45, -70.8206) -> (105.593, -70.9159)
  line L1561 (91.7839, -70.9159) -> (91.9268, -70.8206)
  line L1562 (91.9286, -72.0155) -> (91.9717, -72.073)
  line L1563 (91.9286, -71.2087) -> (91.8743, -71.3536)
  line L1564 (91.9315, -70.819) -> (91.935, -70.8155)
  line L1565 (92.36, -71.8706) -> (92.36, -71.3536)
  line L1566 (92.36, -71.3536) -> (92.3056, -71.2087)
  line L1567 (105.442, -70.8155) -> (105.446, -70.819)
  line L1568 (92.0003, -72.4284) -> (91.968, -72.4175)
  line L1569 (91.9268, -70.8206) -> (91.9315, -70.819)
  line L1570 (92.0052, -70.7967) -> (92.01, -70.7954)
  line L1571 (91.7671, -70.935) -> (91.7839, -70.9159)
  line L1572 (91.9717, -71.1512) -> (91.9286, -71.2087)
  line L1573 (91.8743, -71.8706) -> (91.9286, -72.0155)
  line L1574 (105.372, -70.7967) -> (105.377, -70.7957)
  line L1575 (92.2243, -70.7954) -> (92.229, -70.7967)
  line L1576 (92.1788, -72.1288) -> (92.2625, -72.073)
  line L1577 (105.377, -70.7957) -> (105.409, -70.8067)
  line L1578 (105.731, -71.2311) -> (105.731, -71.4216)
  line L1579 (105.726, -71.4606) -> (105.716, -71.4776)
  line L1580 (105.65, -70.988) -> (105.722, -71.1785)
  line L1581 (144.445, -81.334) -> (144.507, -81.3)
  line L1582 (142.182, -91.3939) -> (142.144, -91.3422)
  line L1583 (105.637, -71.5567) -> (105.62, -71.5666)
  line L1584 (142.157, -83.626) -> (142.174, -83.605)
  line L1585 (105.644, -70.9742) -> (105.646, -70.9817)
  line L1586 (144.879, -81.773) -> (144.882, -81.7771)
  line L1587 (144.578, -81.3051) -> (144.635, -81.3476)
  line L1588 (105.576, -72.0491) -> (105.635, -72.1003)
  line L1589 (105.656, -71.5515) -> (105.637, -71.5567)
  line L1590 (105.409, -72.4175) -> (105.377, -72.4284)
  line L1591 (104.998, -72.4036) -> (104.855, -72.3083)
  line L1592 (105.697, -71.5106) -> (105.687, -71.5278)
  line L1593 (104.843, -72.2994) -> (104.825, -72.2737)
  line L1594 (104.803, -72.2425) -> (104.798, -72.2362)
  line L1595 (105.127, -72.1288) -> (105.322, -72.1288)
  line L1596 (105.711, -71.4966) -> (105.697, -71.5106)
  line L1597 (105.605, -70.9248) -> (105.624, -70.9505)
  line L1598 (105.593, -72.3083) -> (105.45, -72.4036)
  line L1599 (104.804, -72.25) -> (104.803, -72.2425)
  line L1600 (142.453, -91.6965) -> (142.434, -91.6719)
  line L1601 (142.181, -91.395) -> (142.182, -91.3939)
  line L1602 (105.66, -72.1739) -> (105.644, -72.25)
  line L1603 (104.825, -72.2737) -> (104.804, -72.25)
  line L1604 (105.322, -72.1288) -> (105.427, -72.0587)
  line L1605 (104.717, -71.2311) -> (104.724, -71.2052)
  line L1606 (105.427, -72.0587) -> (105.5, -72.0338)
  line L1607 (105.062, -72.0856) -> (105.127, -72.1288)
  line L1608 (104.798, -72.2362) -> (104.727, -72.0457)
  line L1609 (104.717, -71.993) -> (104.717, -71.2311)
  line L1610 (105.003, -72.4052) -> (104.998, -72.4036)
  line L1611 (105.367, -72.4288) -> (105.081, -72.4288)
  line L1612 (105.624, -70.9505) -> (105.644, -70.9742)
  line L1613 (105.722, -71.1785) -> (105.724, -71.2052)
  line L1614 (105.646, -70.9817) -> (105.65, -70.988)
  line L1615 (105.006, -72.4087) -> (105.003, -72.4052)
  line L1616 (105.62, -71.5666) -> (105.017, -71.7273)
  line L1617 (105.039, -72.4175) -> (105.006, -72.4087)
  line L1618 (104.855, -72.3083) -> (104.85, -72.3025)
  line L1619 (105.077, -72.4275) -> (105.072, -72.4284)
  line L1620 (105.017, -71.9658) -> (105.062, -72.0856)
  line L1621 (105.635, -72.1003) -> (105.66, -72.1739)
  line L1622 (104.727, -72.0457) -> (104.724, -72.019)
  line L1623 (105.593, -70.9159) -> (105.598, -70.9216)
  line L1624 (105.644, -72.25) -> (105.593, -72.3083)
  line L1625 (105.446, -72.4052) -> (105.442, -72.4087)
  line L1626 (105.687, -71.5278) -> (105.67, -71.5376)
  line L1627 (105.598, -70.9216) -> (105.605, -70.9248)
  line L1628 (105.081, -72.4288) -> (105.077, -72.4275)
  line L1629 (105.377, -72.4284) -> (105.372, -72.4275)
  line L1630 (105.072, -72.4284) -> (105.039, -72.4175)
  line L1631 (105.442, -72.4087) -> (105.409, -72.4175)
  line L1632 (105.45, -72.4036) -> (105.446, -72.4052)
  line L1633 (144.882, -81.7771) -> (144.886, -81.7808)
  line L1634 (144.886, -81.7808) -> (144.886, -81.7808)
  line L1635 (104.85, -72.3025) -> (104.843, -72.2994)
  line L1636 (105.372, -72.4275) -> (105.367, -72.4288)
  line L1637 (142.334, -91.5379) -> (142.331, -91.5333)
  line L1638 (105.726, -71.4408) -> (105.726, -71.4606)
  line L1639 (105.5, -72.0338) -> (105.576, -72.0491)
  line L1640 (104.724, -72.019) -> (104.717, -71.993)
  line L1641 (144.986, -81.8869) -> (145.055, -81.9594)
  line L1642 (142.599, -92.0811) -> (142.598, -92.0753)
  line L1643 (107.758, -70.1377) -> (107.791, -70.1446)
  line L1644 (142.137, -83.6941) -> (142.157, -83.626)
  line L1645 (104.855, -70.9159) -> (104.998, -70.8206)
  line L1646 (104.804, -70.9742) -> (104.825, -70.9505)
  line L1647 (144.507, -81.3) -> (144.578, -81.3051)
  line L1648 (105.387, -71.1386) -> (105.322, -71.0954)
  line L1649 (104.843, -70.9248) -> (104.85, -70.9216)
  line L1650 (144.879, -81.773) -> (144.879, -81.773)
  line L1651 (104.998, -70.8206) -> (105.003, -70.819)
  line L1652 (107.59, -70.2117) -> (107.593, -70.2082)
  line L1653 (105.062, -71.1386) -> (105.017, -71.2583)
  line L1654 (107.72, -70.13) -> (107.724, -70.1288)
  line L1655 (142.532, -91.8577) -> (142.455, -91.7017)
  line L1656 (104.798, -70.988) -> (104.803, -70.9817)
  line L1657 (144.886, -81.7808) -> (144.986, -81.8869)
  line L1658 (142.455, -91.7017) -> (142.453, -91.6965)
  line L1659 (142.543, -91.8792) -> (142.532, -91.8577)
  line L1660 (107.574, -72.1288) -> (107.574, -70.824)
  line L1661 (105.003, -70.819) -> (105.006, -70.8155)
  line L1662 (105.017, -71.2583) -> (105.017, -71.4169)
  line L1663 (105.431, -71.2583) -> (105.387, -71.1386)
  line L1664 (107.795, -70.1477) -> (107.799, -70.1489)
  line L1665 (107.334, -70.6444) -> (107.453, -70.4853)
  line L1666 (107.574, -70.824) -> (107.559, -70.845)
  line L1667 (105.081, -70.7954) -> (105.367, -70.7954)
  line L1668 (142.174, -83.605) -> (144.445, -81.334)
  line L1669 (142.144, -91.3422) -> (142.137, -91.2996)
  line L1670 (144.744, -81.5739) -> (144.744, -81.5739)
  line L1671 (105.322, -71.0954) -> (105.127, -71.0954)
  line L1672 (107.146, -72.2788) -> (107.166, -72.2038)
  line L1673 (105.072, -70.7957) -> (105.077, -70.7967)
  line L1674 (142.434, -91.6719) -> (142.334, -91.5379)
  line L1675 (105.431, -71.3064) -> (105.431, -71.2583)
  line L1676 (105.077, -70.7967) -> (105.081, -70.7954)
  line L1677 (105.039, -70.8067) -> (105.072, -70.7957)
  line L1678 (144.741, -81.5697) -> (144.744, -81.5739)
  line L1679 (105.006, -70.8155) -> (105.039, -70.8067)
  line L1680 (105.127, -71.0954) -> (105.062, -71.1386)
  line L1681 (105.017, -71.4169) -> (105.431, -71.3064)
  line L1682 (105.367, -70.7954) -> (105.372, -70.7967)
  line L1683 (107.166, -72.2038) -> (107.221, -72.1489)
  line L1684 (107.166, -72.3538) -> (107.146, -72.2788)
  line L1685 (104.724, -71.2052) -> (104.727, -71.1785)
  line L1686 (144.635, -81.3476) -> (144.648, -81.3699)
  line L1687 (142.598, -92.0753) -> (142.543, -91.8792)
  line L1688 (142.137, -91.2996) -> (142.137, -83.6941)
  line L1689 (144.744, -81.5739) -> (144.879, -81.773)
  line L1690 (104.825, -70.9505) -> (104.843, -70.9248)
  line L1691 (107.221, -72.4087) -> (107.166, -72.3538)
  line L1692 (104.727, -71.1785) -> (104.798, -70.988)
  line L1693 (107.221, -72.1489) -> (107.296, -72.1288)
  line L1694 (104.85, -70.9216) -> (104.855, -70.9159)
  line L1695 (107.296, -72.1288) -> (107.574, -72.1288)
  line L1696 (107.593, -70.2082) -> (107.594, -70.2038)
  line L1697 (107.715, -70.129) -> (107.72, -70.13)
  line L1698 (142.334, -91.5379) -> (142.334, -91.5379)
  line L1699 (107.619, -70.1794) -> (107.642, -70.1536)
  line L1700 (104.803, -70.9817) -> (104.804, -70.9742)
  line L1701 (107.683, -70.1399) -> (107.715, -70.129)
  line L1702 (144.648, -81.3699) -> (144.728, -81.5403)
  line L1703 (142.331, -91.5333) -> (142.181, -91.395)
  line L1704 (144.728, -81.5403) -> (144.741, -81.5697)
  line L1705 (88.3717, -70.7273) -> (88.4431, -71.1083)
  line L1706 (88.4431, -71.4493) -> (88.3717, -71.8302)
  line L1707 (87.8258, -70.1368) -> (87.8566, -70.1417)
  line L1708 (88.3717, -71.8302) -> (88.366, -71.8421)
  line L1709 (107.379, -70.975) -> (107.305, -70.9999)
  line L1710 (88.3647, -70.7023) -> (88.366, -70.7154)
  line L1711 (88.3647, -71.8552) -> (88.2933, -72.0457)
  line L1712 (107.724, -70.1288) -> (107.758, -70.1377)
  line L1713 (107.851, -70.2005) -> (107.854, -70.2038)
  line L1714 (107.873, -70.2743) -> (107.874, -70.2788)
  line L1715 (107.559, -70.845) -> (107.539, -70.8607)
  line L1716 (88.2728, -70.4745) -> (88.2808, -70.4944)
  line L1717 (108.153, -72.1288) -> (108.228, -72.1489)
  line L1718 (107.146, -70.8598) -> (107.161, -70.7837)
  line L1719 (107.874, -70.2788) -> (107.874, -72.1288)
  line L1720 (107.646, -70.1521) -> (107.649, -70.1489)
  line L1721 (88.366, -70.7154) -> (88.3717, -70.7273)
  line L1722 (88.1003, -70.2607) -> (88.13, -70.284)
  line L1723 (87.9134, -72.0623) -> (88.0199, -71.9202)
  line L1724 (87.8258, -72.4207) -> (87.7957, -72.4288)
  line L1725 (107.171, -70.9334) -> (107.146, -70.8598)
  line L1726 (107.161, -70.7837) -> (107.212, -70.7254)
  line L1727 (107.874, -70.2698) -> (107.873, -70.2743)
  line L1728 (107.453, -70.4853) -> (107.59, -70.2117)
  line L1729 (107.229, -70.9847) -> (107.171, -70.9334)
  line L1730 (107.522, -70.8798) -> (107.379, -70.975)
  line L1731 (107.824, -70.1732) -> (107.849, -70.1961)
  line L1732 (88.2933, -70.5118) -> (88.3647, -70.7023)
  line L1733 (88.4457, -71.1359) -> (88.4457, -71.4216)
  line L1734 (88.4431, -71.1083) -> (88.442, -71.1223)
  line L1735 (88.2808, -70.4944) -> (88.2933, -70.5118)
  line L1736 (88.13, -70.284) -> (88.2728, -70.4745)
  line L1737 (107.863, -70.2371) -> (107.874, -70.2698)
  line L1738 (108.283, -72.2038) -> (108.303, -72.2788)
  line L1739 (107.791, -70.1446) -> (107.795, -70.1477)
  line L1740 (107.874, -72.1288) -> (108.153, -72.1288)
  line L1741 (108.228, -72.1489) -> (108.283, -72.2038)
  line L1742 (107.212, -70.7254) -> (107.334, -70.6444)
  line L1743 (107.799, -70.1489) -> (107.824, -70.1732)
  line L1744 (87.8566, -70.1417) -> (88.0709, -70.2369)
  line L1745 (108.153, -72.4288) -> (107.296, -72.4288)
  line L1746 (107.649, -70.1489) -> (107.683, -70.1399)
  line L1747 (107.594, -70.2038) -> (107.619, -70.1794)
  line L1748 (88.366, -71.8421) -> (88.3647, -71.8552)
  line L1749 (108.283, -72.3538) -> (108.228, -72.4087)
  line L1750 (108.228, -72.4087) -> (108.153, -72.4288)
  line L1751 (108.303, -72.2788) -> (108.283, -72.3538)
  line L1752 (107.854, -70.2038) -> (107.863, -70.2371)
  line L1753 (107.539, -70.8607) -> (107.522, -70.8798)
  line L1754 (107.296, -72.4288) -> (107.221, -72.4087)
  line L1755 (107.642, -70.1536) -> (107.646, -70.1521)
  line L1756 (107.305, -70.9999) -> (107.229, -70.9847)
  line L1757 (88.0709, -70.2369) -> (88.1003, -70.2607)
  line L1758 (107.849, -70.1961) -> (107.851, -70.2005)
  line L1759 (88.4457, -71.4216) -> (88.442, -71.4352)
  line L1760 (88.442, -71.4352) -> (88.4431, -71.4493)
  line L1761 (88.442, -71.1223) -> (88.4457, -71.1359)
  line L1762 (141.394, -80.7524) -> (141.225, -80.6462)
  line L1763 (144.939, -79.0437) -> (144.922, -79.0646)
  line L1764 (144.406, -72.3395) -> (144.408, -72.3445)
  line L1765 (141.802, -81.8899) -> (141.803, -81.8629)
  line L1766 (144.622, -71.0999) -> (144.622, -71.0999)
  line L1767 (144.349, -71.688) -> (144.329, -71.9074)
  line L1768 (141.543, -80.8907) -> (141.394, -80.7524)
  line L1769 (141.178, -80.5929) -> (141.167, -80.5396)
  line L1770 (141.647, -81.0293) -> (141.547, -80.8953)
  line L1771 (144.329, -71.9074) -> (144.349, -72.1268)
  line L1772 (141.345, -72.8751) -> (141.501, -72.7194)
  line L1773 (141.828, -81.6939) -> (141.829, -81.6356)
  line L1774 (141.803, -81.8629) -> (141.805, -81.8497)
  line L1775 (141.547, -80.8953) -> (141.547, -80.8953)
  line L1776 (141.167, -73.0658) -> (141.187, -72.9976)
  line L1777 (144.622, -71.0999) -> (144.528, -71.2339)
  line L1778 (141.755, -81.2366) -> (141.745, -81.2151)
  line L1779 (144.625, -72.7194) -> (144.781, -72.8751)
  line L1780 (141.955, -82.0041) -> (141.884, -81.999)
  line L1781 (144.959, -73.0658) -> (144.959, -78.9755)
  line L1782 (144.502, -72.5436) -> (144.502, -72.5436)
  line L1783 (144.499, -72.5391) -> (144.502, -72.5436)
  line L1784 (144.406, -71.4753) -> (144.349, -71.688)
  line L1785 (144.781, -72.8751) -> (144.785, -72.8783)
  line L1786 (144.408, -72.3445) -> (144.496, -72.5341)
  line L1787 (144.496, -72.5341) -> (144.499, -72.5391)
  line L1788 (141.341, -72.8783) -> (141.341, -72.8783)
  line L1789 (144.959, -78.9755) -> (144.939, -79.0437)
  line L1790 (144.922, -79.0646) -> (142.017, -81.97)
  line L1791 (144.455, -71.3702) -> (144.406, -71.4753)
  line L1792 (144.499, -71.2757) -> (144.496, -71.2807)
  line L1793 (141.624, -72.5436) -> (141.624, -72.5436)
  line L1794 (141.827, -81.9564) -> (141.802, -81.8899)
  line L1795 (141.627, -72.5391) -> (141.629, -72.5341)
  line L1796 (141.341, -72.8783) -> (141.345, -72.8751)
  line L1797 (141.829, -81.6356) -> (141.811, -81.4327)
  line L1798 (144.528, -71.2339) -> (144.499, -71.2757)
  line L1799 (141.287, -72.9157) -> (141.341, -72.8783)
  line L1800 (144.502, -72.5436) -> (144.595, -72.6768)
  line L1801 (144.95, -73.018) -> (144.959, -73.0658)
  line L1802 (144.349, -72.1268) -> (144.406, -72.3395)
  line L1803 (144.906, -72.9625) -> (144.95, -73.018)
  line L1804 (141.665, -81.0539) -> (141.647, -81.0293)
  line L1805 (142.017, -81.97) -> (141.955, -82.0041)
  line L1806 (144.496, -72.5341) -> (144.496, -72.5341)
  line L1807 (141.501, -72.7194) -> (141.531, -72.6768)
  line L1808 (144.839, -72.9157) -> (144.906, -72.9625)
  line L1809 (144.496, -71.2807) -> (144.496, -71.2807)
  line L1810 (141.547, -80.8953) -> (141.543, -80.8907)
  line L1811 (141.531, -72.6768) -> (141.624, -72.5436)